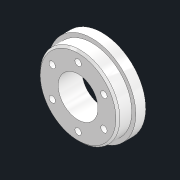
# Autodesk Inventor part: base1
Saved by Autodesk Inventor 2021 (Build 250183000, 183)
## iProperties
Created: 2021-07-30
Part Number: base1
Material: ABS プラスチック
Document SubType Name: Modeling
Designer: yuta0
Density: 1.06 g/cm^3
Appearance: 滑らか - 白
Mass: 12.7077 g
Surface Area: 52.8992 cm^2
Volume: 11.9884 cm^3
Author: yuta0
Autodesk Inventor part; units mm, degrees
ref_plane "YZ Plane" through (0, 0, 0) normal (1, 0, 0) x (0, 1, 0)
ref_plane "XZ Plane" through (0, 0, 0) normal (0, 1, 0) x (-1, 0, 0)
ref_plane "XY Plane" through (0, 0, 0) normal (0, 0, 1) x (1, 0, 0)
sketch "スケッチ1" plane through (0, 0, 0) normal (1, 0, 0) x (0, 1, 0)
  line L0 (10, 0) -> (10, -12)
  line L1 (22, -12) -> (22, -7)
  line L2 (22, -7) -> (20, -7)
  line L3 (20, -7) -> (20, 0)
  line L4 (20, 0) -> (10, 0)
  line L5 (0, -14.4) -> (0, 2.4) projected
  line L6 (22, -12) -> (10, -12)
  point P0 (0, 0)
  dimension "d0" = 20
  dimension "d1" = 2
  dimension "d2" = 7
  dimension "d3" = 5
  dimension "d4" = 10
  constraints: 12 end point, 5 perpendicular, 1 horizontal alignment, 1 vertical
  measures "d0" distance from line of point (0, 0) L3
  measures "d1" distance of L1.end L2.end
  measures "d2" distance of L2.end L3.end
  measures "d3" distance of L1.start L1.end
  measures "d4" distance of L3.end L0.start
revolve "回転1" add sketch "スケッチ1" angle 360 about axis through (0, 0, -10) along (0, 0, 1)
sketch "スケッチ2" plane through (0, 0, 0) normal (0, 0, 1) x (1, 0, 0)
  circle A0 centre (0, 0) radius 20 projected
  circle A1 centre (0, 0) radius 15
  point P0 (0, 15)
  point P1 (-12.9904, 7.5)
  point P2 (-12.9904, -7.5)
  point P3 (0, -15)
  point P4 (12.9904, -7.5)
  point P5 (12.9904, 7.5)
  dimension "d8" = 5
  dimension "d11" = 360
  constraints: 1 vertical alignment, 9 other
hole "穴1" at (0, 15, 0) at (-12.9904, 7.5, 0) at (-12.9904, -7.5, 0) at (0, -15, 0) at (12.9904, -7.5, 0) at (12.9904, 7.5, 0) direction (0, 0, -1) diameter 3.2 end through all clearance for "Socket Head Cap Screw" size "M3" standard "Ansi Metric M Profile"
chamfer "面取り1" distance 1 angle 45 1 edges at (0, -20, 0)
